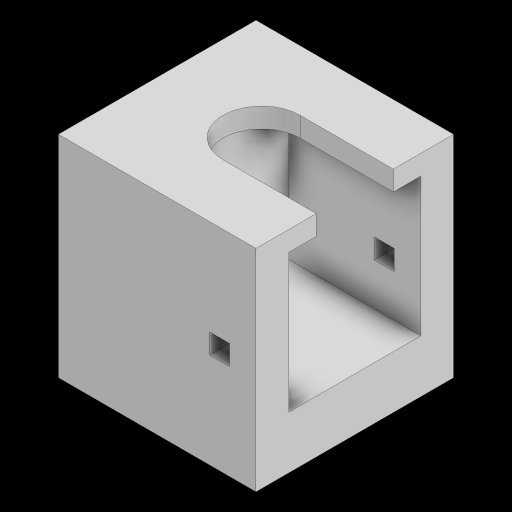
# Autodesk Inventor part: valve_mount
Saved by Autodesk Inventor 2023 (Build 270158000, 158)
## iProperties
Created: 2024-07-04
Part Number: valve_mount
Material: 일반
Document SubType Name: Modeling
Designer: OMS55
Density: 1 g/cm^3
Appearance: 기본값
Author: OMS55
Autodesk Inventor part; units mm, degrees
ref_plane "YZ Plane" through (0, 0, 0) normal (1, 0, 0) x (0, 1, 0)
ref_plane "XZ Plane" through (0, 0, 0) normal (0, 1, 0) x (-1, 0, 0)
ref_plane "XY Plane" through (0, 0, 0) normal (0, 0, 1) x (1, 0, 0)
sketch "스케치2" plane through (0, 0, 0) normal (0, 1, 0) x (-1, 0, 0)
  line L0 (0, 0) -> (-30, 0)
  line L1 (-30, 0) -> (-30, -30)
  line L2 (-30, -30) -> (0, -30)
  line L3 (0, -30) -> (0, 0)
  line L4 (-10, -5) -> (-30, -5)
  line L5 (-30, -5) -> (-30, -25)
  line L6 (-30, -25) -> (-10, -25)
  line L7 (-10, -25) -> (-10, -5)
  point P0 (0, -15)
  point P1 (-10, -15)
  dimension "d0" = 30
  dimension "d1" = 30
  dimension "d2" = 20
  dimension "d3" = 20
  constraints: 16 end point, 4 parallel, 2 horizontal, 2 midpoint, 2 perpendicular, 1 coincident, 1 collinear, 1 horizontal alignment
  measures "d0" distance of L2.end L0.start
  measures "d1" distance of L1.end L2.end
  measures "d2" distance of L6.end L4.start
  measures "d3" distance of L5.end L6.end
extrude "돌출1" add sketch "스케치2" along normal blind 32 contours L3 L2 L1 L6 L7 L4 L0
sketch "스케치3" plane through (0, 0, -30) normal (-1, 0, 0) x (0, 0, 1)
  circle A0 centre (15, 14.6) radius 6.75
  line L0 (0, 32) -> (30, 32)
  line L1 (30, 0) -> (30, 32)
  line L2 (0, 0) -> (30, 0) projected
  point P0 (15, 32)
  point P1 (30, 16)
  dimension "d6" = 13.5
  dimension "d34" = 14.6
  constraints: 4 end point, 2 midpoint, 1 centre point
  measures "d6" diameter of A0
  measures "d34" distance from line of L2 A0.centre
extrude "돌출2" cut sketch "스케치3" against normal blind 20
sketch "스케치4" plane through (10, 0, -5) normal (1, 0, 0) x (0, 0, -1)
  line L0 (0, 32) -> (20, 32)
  line L1 (20, 32) -> (20, 29)
  line L2 (20, 29) -> (0, 29)
  line L3 (0, 29) -> (0, 32)
  line L4 (0, 32) -> (20, 32) projected
  circle A0 centre (10, 14.6) radius 6.75 projected
  line L5 (0, 0) -> (0, 32) projected
  point P0 (-5, 0)
  point P1 (10, 32)
  point P2 (10, 32)
  dimension "d10" = 3
  dimension "d11" = 17.4
  constraints: 8 end point, 2 midpoint, 2 parallel, 1 coincident, 1 collinear, 1 horizontal, 1 perpendicular
  measures "d10" distance of L0.end L1.end
  measures "d11" distance from line of L0 A0.centre
extrude "돌출3" add sketch "스케치4" along normal up to surface (20 mm away) contours L0 L1 L2 L3
sketch "스케치6" plane through (0, 32, 0) normal (0, 1, 0) x (1, 0, 0)
  line L0 (15.85, 15) -> (69.8483, 15) construction
  line L1 (15.85, 9.15) -> (69.8483, 9.15)
  line L2 (69.8483, 20.85) -> (15.85, 20.85)
  arc A0 (15.85, 20.85) -> (15.85, 9.15) centre (15.85, 15) ccw
  arc A1 (69.8483, 9.15) -> (69.8483, 20.85) centre (69.8483, 15) ccw
  line L3 (30, 0) -> (30, 30) projected
  line L4 (0, 30) -> (0, 0) projected
  point P0 (42.8492, 15)
  point P1 (10, 15)
  point P2 (30, 15)
  point P3 (30, 9.15)
  point P4 (30, 20.85)
  dimension "d19" = 11.7
  dimension "d20" = 10
  constraints: 8 end point, 5 point on circle, 4 tangent, 2 centre point, 2 midpoint, 1 horizontal, 1 horizontal alignment, 1 parallel
  measures "d19" distance between parallel lines of L1 L2
  measures "d20" distance from line of point (10, 15) L4
extrude "돌출5" cut sketch "스케치6" against normal blind 28 contours A0 L2 L3 L1
sketch "스케치7" plane through (10, 0, -5) normal (1, 0, 0) x (0, 0, -1)
  line L0 (0, 8) -> (20, 8)
  line L1 (20, 8) -> (20, 0)
  line L2 (20, 0) -> (0, 0)
  line L3 (0, 0) -> (0, 8)
  circle A0 centre (10, 14.6) radius 6.75 projected
  point P0 (-5, 0)
  dimension "d32" = 8
  dimension "d33" = 8
  constraints: 8 end point, 2 coincident, 1 parallel
  measures "d32" distance of L2.end L0.start
  measures "d33" distance of L0.end L1.end
extrude "돌출6" add sketch "스케치7" along normal up to surface (20 mm away) contours L0 A0 L1 L2 L3 | L0 A0 picked at (10.1583, 7.9556)
sketch "스케치8" plane through (30, 0, -30) normal (0, 0, -1) x (-1, 0, 0)
  line L0 (30, 0) -> (30, 32) projected
  line L1 (4, 17.5) -> (7, 17.5)
  line L2 (7, 17.5) -> (7, 14.5)
  line L3 (7, 14.5) -> (4, 14.5)
  line L4 (4, 14.5) -> (4, 17.5)
  point P0 (7, 16)
  point P1 (30, 16)
  dimension "d27" = 23
  dimension "d28" = 3
  dimension "d29" = 3
  constraints: 8 end point, 2 midpoint, 2 parallel, 1 horizontal, 1 horizontal alignment, 1 perpendicular
  measures "d27" distance between parallel lines of L0 L2
  measures "d28" distance of L1.start L1.end
  measures "d29" distance of L1.end L2.end
extrude "돌출7" cut sketch "스케치8" against normal blind 40
